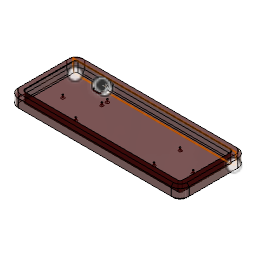
PlanckHiProCase (Autodesk Fusion 360 design; units mm, degrees)
part number: 2025-12-26-20-35-43-522
Autodesk Fusion 360 part; units mm, degrees
note: some values were not read from the file. Set by a fixed rule: which sketch regions a step uses.
ref_plane "WorkPlane1" through (0, 0, -6) normal (0, 0, 1) x (1, 0, 0)
ref_plane "WorkPlane2" through (0, 0, -5) normal (0, 0, 1) x (1, 0, 0)
other "Base Mesh Feature2"
sketch "Walls" plane through (0, 0, -6) normal (0, 0, 1) x (1, 0, 0)
  line L0 (111.325, 38.5) -> (-111.325, 38.5)
  arc A0 (114.5, 35.325) -> (111.325, 38.5) centre (111.325, 35.325) ccw
  line L1 (114.5, -35.325) -> (114.5, 35.325)
  arc A1 (111.325, -38.5) -> (114.5, -35.325) centre (111.325, -35.325) ccw
  line L2 (-111.325, -38.5) -> (111.325, -38.5)
  arc A2 (-114.5, -35.325) -> (-111.325, -38.5) centre (-111.325, -35.325) ccw
  line L3 (-114.5, 35.325) -> (-114.5, -35.325)
  arc A3 (-111.325, 38.5) -> (-114.5, 35.325) centre (-111.325, 35.325) ccw
  line L4 (-124.5, 35.325) -> (-124.5, -35.325)
  arc A4 (-124.5, -35.325) -> (-111.325, -48.5) centre (-111.325, -35.325) ccw
  line L5 (-111.325, -48.5) -> (111.325, -48.5)
  arc A5 (111.325, -48.5) -> (124.5, -35.325) centre (111.325, -35.325) ccw
  line L6 (124.5, -35.325) -> (124.5, 35.325)
  arc A6 (124.5, 35.325) -> (111.325, 48.5) centre (111.325, 35.325) ccw
  line L7 (111.325, 48.5) -> (-111.325, 48.5)
  arc A7 (-111.325, 48.5) -> (-124.5, 35.325) centre (-111.325, 35.325) ccw
  dimension "d23" = 38.5
  dimension "d24" = 38.5
  dimension "d25" = 114.5
  dimension "d26" = 114.5
  dimension "d28" = 3.175
  dimension "d29" = 10
  constraint horizontal L2
  constraint horizontal L0
  constraint tangent L2 A2
  constraint tangent A1 L2
  constraint tangent L0 A0
  constraint tangent L0 A3
  constraint tangent A2 L3
  constraint vertical L3
  constraint vertical L1
  constraint tangent L1 A1
  constraint tangent A0 L1
  constraint tangent L3 A3
  constraint coincident L3.start A3.end
  constraint equal A2 A3
  constraint equal A1 A3
  constraint equal A0 A3
  measures "d23" distance of origin L0
  measures "d24" distance of origin L2
  measures "d25" distance of origin L3
  measures "d26" distance of origin L1
  measures "d28" radius of A3
other "MeshSection2"
ref_plane "WorkPlane3" through (0, 38.5, 0) normal (0, 1, 0) x (0, 0, 1)
sketch "Floor" plane through (0, 0, -5) normal (0, 0, 1) x (1, 0, 0)
  circle A0 centre (-95, -0.0001) radius 1.0986
  circle A1 centre (-56.999, 27.0014) radius 0.9987
  circle A2 centre (-57, 18.9999) radius 1.0986
  circle A3 centre (-57, -19) radius 1.0985
  circle A4 centre (57, -19) radius 1.0985
  circle A5 centre (57, 18.9999) radius 1.0986
  circle A6 centre (95, -0.0001) radius 1.0986
  line L0 (-81.249, 38.5014) -> (-81.249, 29.0014)
  line L1 (-81.249, 29.0014) -> (-70.749, 29.0014)
  line L2 (-70.749, 29.0014) -> (-70.749, 38.5014)
  line L3 (-81.249, 38.5014) -> (-70.749, 38.5014)
  dimension "d10" = 10.5
  dimension "d21" = 2
  dimension "d22" = 13.75
  dimension "d56" = 11.5
  constraint horizontal L1
  constraint vertical L0
  constraint vertical L2
  constraint coincident L0.end L1.start
  constraint coincident L1.end L2.start
  measures "d10" distance of L0 L2
  measures "d21" distance of A1.centre L1
  measures "d22" distance of A1.centre L2
  measures "d56" distance of A1.centre L3
other "MeshSection1"
extrude "Extrude1" add sketch "Walls" against normal blind 4 contours L0 A0 L1 A1 L2 A2 L3 A3 | L4 A4 L5 A5 L6 A6 L7 A7
extrude "Extrude2" add sketch "Walls" along normal blind 15
chamfer "Chamfer1" distance 0.5 angle 45 8 edges at (-113.5701, 37.5701, 9) (0, 38.5, 9) (113.5701, 37.5701, 9) (114.5, 0, 9) (113.5701, -37.5701, 9) (0, -38.5, 9) (-113.5701, -37.5701, 9) (-114.5, 0, 9)
chamfer "Chamfer1" distance 3.3333 angle 45 16 edges at (0, 48.5, 9) (-120.6411, 44.6411, 9) (-124.5, 0, 9) (-120.6411, -44.6411, 9) (0, -48.5, 9) (120.6411, -44.6411, 9) (124.5, 0, 9) (120.6411, 44.6411, 9) (0, 48.5, -10) (120.6411, 44.6411, -10) (124.5, 0, -10) (120.6411, -44.6411, -10) (0, -48.5, -10) (-120.6411, -44.6411, -10) (-124.5, 0, -10) (-120.6411, 44.6411, -10)
sketch "BackInnerCutout" plane through (0, 38.5, 0) normal (0, 1, 0) x (-1, 0, 0)
  line L0 (70.75, -5.1584) -> (70.75, -5.9834)
  line L1 (79.6625, -3.5709) -> (72.3375, -3.5709)
  line L2 (72.3375, -7.5709) -> (79.6625, -7.5709)
  line L3 (115.5, -9.0709) -> (70.75, -9.0709) construction
  line L4 (-115.5, -9.0709) -> (70.75, -9.0709) construction
  line L5 (81.25, -5.1584) -> (81.25, -5.9834)
  arc A0 (72.3375, -3.5709) -> (70.75, -5.1584) centre (72.3375, -5.1584) ccw
  arc A1 (81.25, -5.1584) -> (79.6625, -3.5709) centre (79.6625, -5.1584) ccw
  arc A2 (79.6625, -7.5709) -> (81.25, -5.9834) centre (79.6625, -5.9834) ccw
  arc A3 (70.75, -5.9834) -> (72.3375, -7.5709) centre (72.3375, -5.9834) ccw
  point P0 (76, -3.5709)
  dimension "d39" = 5.25
  dimension "d40" = 5.25
  dimension "d53" = 1.5875
  dimension "d59" = 1.5
  dimension "d60" = 4
  constraint horizontal L1
  constraint vertical L0
  constraint horizontal L2
  constraint vertical L5
  constraint coincident L1 P0
  constraint tangent L0 A0
  constraint tangent L1 A0
  constraint tangent L1 A1
  constraint tangent L5 A1
  constraint equal A0 A1
  constraint tangent L5 A2
  constraint tangent L2 A2
  constraint equal A0 A2
  constraint tangent L2 A3
  constraint tangent L0 A3
  constraint equal A0 A3
  constraint horizontal L4
  constraint horizontal L3
  measures "d39" distance of P0 L5
  measures "d40" distance of L0 P0
  measures "d53" radius of A0
  measures "d59" distance of L2 L3
  measures "d60" distance of L1 L2
other "MeshSection3"
extrude "USBCutBack" cut sketch "BackInnerCutout" along normal through all
ref_plane "WorkPlane4" through (0, 41, 1.5) normal (0, -1, 0) x (1, 0, 0)
sketch "BackOuterCutout" plane through (0, 41, 0) normal (0, -1, 0) x (-1, 0, 0)
  line L0 (81.25, 5.1584) -> (81.25, 5.9834)
  arc A0 (79.6625, 3.5709) -> (81.25, 5.1584) centre (79.6625, 5.1584) ccw
  line L1 (79.6625, 3.5709) -> (72.3375, 3.5709)
  arc A1 (70.75, 5.1584) -> (72.3375, 3.5709) centre (72.3375, 5.1584) ccw
  line L2 (70.75, 5.1584) -> (70.75, 5.9834)
  arc A2 (72.3375, 7.5709) -> (70.75, 5.9834) centre (72.3375, 5.9834) ccw
  arc A3 (81.25, 5.9834) -> (79.6625, 7.5709) centre (79.6625, 5.9834) ccw
  line L3 (72.3375, 7.5709) -> (79.6625, 7.5709)
  arc A4 (69.75, 5.1584) -> (72.3375, 2.5709) centre (72.3375, 5.1584) ccw
  line L4 (79.6625, 2.5709) -> (72.3375, 2.5709)
  arc A5 (79.6625, 2.5709) -> (82.25, 5.1584) centre (79.6625, 5.1584) ccw
  line L5 (82.25, 5.1584) -> (82.25, 5.9834)
  arc A6 (82.25, 5.9834) -> (79.6625, 8.5709) centre (79.6625, 5.9834) ccw
  line L6 (72.3375, 8.5709) -> (79.6625, 8.5709)
  arc A7 (72.3375, 8.5709) -> (69.75, 5.9834) centre (72.3375, 5.9834) ccw
  line L7 (69.75, 5.1584) -> (69.75, 5.9834)
  dimension "d54" = -1
extrude "Extrude5" cut sketch "BackOuterCutout" against normal through all
extrude "USBCutDown" cut sketch "Floor" against normal blind 2.5709 contours L0 L1 L2 L3
fillet "Fillet4" radius 1.5875 2 edges at (-81.249, 29.0014, -6.7855) (-70.749, 29.0014, -6.7855)
sketch "Holes" plane through (0, 0, -10) normal (0, 0, -1) x (1, 0, 0)
  line L0 (-111.325, -45.1667) -> (111.325, -45.1667)
  arc A0 (111.325, -45.1667) -> (121.1667, -35.325) centre (111.325, -35.325) ccw
  line L1 (121.1667, -35.325) -> (121.1667, 35.325)
  arc A1 (121.1667, 35.325) -> (111.325, 45.1667) centre (111.325, 35.325) ccw
  line L2 (111.325, 45.1667) -> (-111.325, 45.1667)
  arc A2 (-111.325, 45.1667) -> (-121.1667, 35.325) centre (-111.325, 35.325) ccw
  line L3 (-121.1667, 35.325) -> (-121.1667, -35.325)
  arc A3 (-121.1667, -35.325) -> (-111.325, -45.1667) centre (-111.325, -35.325) ccw
  point P0 (57, -18.9999)
  point P1 (95, 0.0001)
  point P2 (57, 19)
  point P3 (-57, 19)
  point P4 (-95, 0.0001)
  point P5 (-57, -18.9999)
  point P6 (-56.999, -27.0014)
hole "Hole1" at (57, -19, -10) at (57, 18.9999, -10) at (95, -0.0001, -10) at (-57, 18.9999, -10) at (-57, -19, -10) at (-95, -0.0001, -10) at (-56.999, 27.0014, -10) direction (0, 0, 1) diameter 2.2 end through all countersink diameter 4.5 countersink angle 90
equation "d4 = -floorThickness"
equation "d26 = d25"
equation "d28 = 1 in / 8"
equation "d29 = wallThickness"
equation "smallFillet = 1 in / 16"
equation "d40 = d39"
equation "wallThickness = 10 mm"
equation "floorThickness = 4 mm"
equation "d47 = wallThickness / 3"
equation "d53 = 1 in / 16"
equation "d58 = smallFillet"
